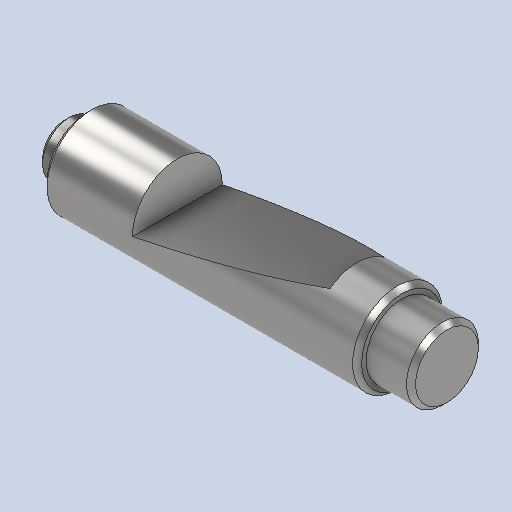
# Autodesk Inventor part: 9-滑轴
Saved by Autodesk Inventor 2022 (Build 260153000, 153)
## iProperties
Created: 2023-01-09
Part Number: 9-滑轴
Material: 不锈钢
Document SubType Name: Modeling
Designer: Lzy18
Density: 8 g/cm^3
Appearance: 半抛光
Author: Lzy18
Autodesk Inventor part; units mm, degrees
ref_plane "YZ Plane" through (0, 0, 0) normal (1, 0, 0) x (0, 1, 0)
ref_plane "XZ Plane" through (0, 0, 0) normal (0, 1, 0) x (-1, 0, 0)
ref_plane "XY Plane" through (0, 0, 0) normal (0, 0, 1) x (1, 0, 0)
sketch "草图1" plane through (0, 0, 0) normal (0, 0, 1) x (1, 0, 0)
  line L0 (0, 0) -> (5, 0)
  line L1 (5, 0) -> (5, -6)
  line L2 (5, -6) -> (0, -6)
  line L3 (0, -6) -> (0, 0)
  line L4 (5, 0) -> (75, 0)
  line L5 (75, 0) -> (75, -10)
  line L6 (75, -10) -> (5, -10)
  line L7 (5, -10) -> (5, 0)
  line L8 (75, 0) -> (85, 0)
  line L9 (85, 0) -> (85, -8)
  line L10 (85, -8) -> (75, -8)
  line L11 (75, -8) -> (75, 0)
  dimension "d0" = 5
  dimension "d1" = 6
  dimension "d2" = 70
  dimension "d3" = 10
  dimension "d4" = 10
  dimension "d5" = 8
  constraints: 24 end point, 6 parallel, 3 horizontal, 3 perpendicular
  measures "d0" distance of L1.end L2.end
  measures "d1" distance of L0.end L1.end
  measures "d2" distance of L5.end L6.end
  measures "d3" distance of L4.end L5.end
  measures "d4" distance of L9.end L10.end
  measures "d5" distance of L8.end L9.end
revolve "旋转1" add sketch "草图1" angle 360 about axis through (5, 0, 0) along (1, 0, 0)
sketch "草图2" plane through (0, 0, 0) normal (0, 0, 1) x (1, 0, 0)
  line L0 (5, 6) -> (0, 6) projected
  line L1 (0, 6) -> (0, -6) projected
  line L2 (1, 6) -> (0, 6)
  line L3 (0, 6) -> (0, 5)
  line L4 (1, 6) -> (0, 5)
  line L5 (1, 6) -> (0, 5)
  line L6 (5, 10) -> (5, -10) projected
  line L7 (5, 10) -> (6, 10)
  line L8 (6, 10) -> (6, 9)
  line L9 (6, 9) -> (5, 9)
  line L10 (5, 9) -> (5, 10)
  line L11 (5, 10) -> (5, 9)
  line L12 (84, 8) -> (84, 7)
  line L13 (84, 7) -> (85, 7)
  line L14 (85, 8) -> (85, -8) projected
  line L15 (85, 8) -> (85, 7)
  line L16 (75, 10) -> (75, -10) projected
  line L17 (75, 10) -> (74, 10)
  line L18 (74, 10) -> (74, 9)
  line L19 (74, 9) -> (75, 9)
  line L20 (75, 9) -> (75, 10)
  line L21 (75, 9) -> (74, 10)
  line L22 (75, 10) -> (75, 9)
  line L23 (85, 8) -> (84, 8)
  line L24 (84, 8) -> (84, 7)
  line L25 (84, 7) -> (85, 7)
  line L26 (85, 7) -> (85, 8)
  line L27 (85, 7) -> (84, 8)
  line L28 (85, 8) -> (85, 7)
  line L29 (6, 10) -> (5, 9)
  line L30 (-17, 0) -> (102, 0) projected
  point P0 (0, 0)
  dimension "d7" = 1
  dimension "d8" = 1
  dimension "d9" = 1
  dimension "d10" = 1
  dimension "d13" = 1
  dimension "d14" = 1
  dimension "d15" = 1
  dimension "d16" = 1
  constraints: 50 end point, 6 parallel, 4 horizontal, 3 collinear, 3 perpendicular, 2 point on line, 2 vertical
  measures "d7" distance from line of L1 L2.start
  measures "d8" distance from line of L0 L3.end
  measures "d9" distance of L8.end L9.end
  measures "d10" distance of L7.end L8.end
  measures "d13" distance of L19.end L18.end
  measures "d14" distance of L18.end L17.end
  measures "d15" distance of L25.end L12.end
  measures "d16" distance of L12.end L23.end
revolve "旋转2" cut sketch "草图2" angle 360 about axis through (-10, 0, 0) along (1, 0, 0) contours L6 L7 L29 | L21 L17 L16 | L27 L23 L14 | L4 L1 L0
sketch "草图3" plane through (0, 0, 0) normal (0, 0, 1) x (1, 0, 0)
  line L0 (74, 10) -> (6, 10) projected
  line L1 (75, 8) -> (75, -8) projected
  line L2 (65, 10) -> (65, 8)
  line L3 (74, 10) -> (74, -10) projected
  line L4 (25, 10) -> (25, 0)
  line L5 (5, 9) -> (5, -9) projected
  line L6 (25, 0) -> (65, 8)
  line L7 (65, 10) -> (25, 10)
  point P0 (0, 0)
  dimension "d18" = 10
  dimension "d19" = 2
  dimension "d20" = 10
  dimension "d21" = 20
  constraints: 8 end point, 2 point on line, 1 horizontal, 1 parallel, 1 vertical
  measures "d18" distance from line of L1 L2.start
  measures "d19" distance of L2.start L2.end
  measures "d20" distance of L4.start L4.end
  measures "d21" distance between parallel lines of L5 L4
extrude "拉伸1" cut sketch "草图3" along normal through all both and the other way through all
